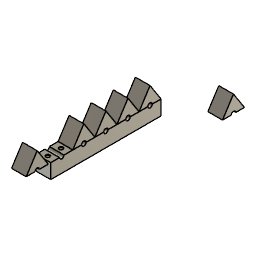
cabel organizer prototype (Autodesk Fusion 360 archive; units mm, degrees)
design "eg project work"
part number: 2025-11-05-01-47-41-680
Autodesk Fusion 360 part; units mm, degrees
sketch "Sketch1" plane through (0, 0, 0) normal (1, 0, 0) x (0, 1, 0)
  line L0 (-100, 50) -> (125, 50)
  line L1 (125, 50) -> (125, 20)
  line L2 (-100, 50) -> (-100, 20)
  line L3 (-100, 20) -> (125, 20)
  dimension "d1" = 225
  dimension "d2" = 30
  dimension "d3" = 30
  constraint horizontal L0
  constraint perpendicular L0 L1
  constraint perpendicular L0 L2
  measures "d1" distance of L0.start L0.end
  measures "d2" distance of L0.end L1.end
  measures "d3" distance of L0.start L2.end
extrude "Extrude1" add sketch "Sketch1" along normal blind 30 makes body 1
sketch "Sketch2" plane through (30, 0, 0) normal (1, 0, 0) x (0, 1, 0)
  line L0 (-100, 50) -> (-100, 20)
  line L1 (-100, 20) -> (125, 20)
  line L2 (125, 20) -> (125, 50)
  line L3 (125, 50) -> (-100, 50)
  circle A0 centre (-91, 50) radius 4
  line L4 (-87, 50) -> (-82, 50)
  circle A1 centre (-77.5, 50) radius 4.5
  line L5 (-73, 50) -> (-68, 50)
  circle A2 centre (-64, 50) radius 4
  line L6 (-60, 50) -> (-50, 50)
  circle A3 centre (-46, 50) radius 4
  line L7 (-42, 50) -> (-37, 50)
  circle A4 centre (-32.5, 50) radius 4.5
  line L8 (-28, 50) -> (-23, 50)
  circle A5 centre (-19.0025, 49.8588) radius 4
  line L9 (-15.005, 50) -> (-5.005, 50)
  circle A6 centre (-1.005, 50) radius 4
  line L10 (2.995, 50) -> (7.995, 50)
  circle A7 centre (12.495, 50) radius 4.5
  line L11 (16.995, 50) -> (21.995, 50)
  circle A8 centre (25.995, 50) radius 4
  line L12 (29.995, 50) -> (34.995, 50)
  line L13 (34.995, 50) -> (39.995, 50)
  circle A9 centre (43.995, 50) radius 4
  line L14 (47.995, 50) -> (52.995, 50)
  circle A10 centre (57.495, 50) radius 4.5
  line L15 (61.995, 50) -> (66.995, 50)
  circle A11 centre (70.995, 50) radius 4
  line L16 (74.995, 50) -> (79.995, 50)
  line L17 (79.995, 50) -> (84.995, 50)
  circle A12 centre (88.995, 50) radius 4
  line L18 (92.995, 50) -> (97.995, 50)
  circle A13 centre (102.495, 50) radius 4.5
  line L19 (106.995, 50) -> (111.995, 50)
  circle A14 centre (115.995, 50) radius 4
  dimension "d6" = 8
  dimension "d7" = 5
  dimension "d8" = 9
  dimension "d9" = 5
  dimension "d10" = 8
  dimension "d11" = 10
  dimension "d12" = 8
  dimension "d13" = 5
  dimension "d14" = 9
  dimension "d15" = 5
  dimension "d16" = 8
  dimension "d17" = 10
  dimension "d18" = 8
  dimension "d19" = 5
  dimension "d20" = 9
  dimension "d21" = 5
  dimension "d22" = 8
  dimension "d23" = 5
  dimension "d24" = 5
  dimension "d25" = 8
  dimension "d26" = 5
  dimension "d27" = 9
  dimension "d28" = 5
  dimension "d29" = 8
  dimension "d30" = 5
  dimension "d31" = 5
  dimension "d32" = 8
  dimension "d33" = 5
  dimension "d34" = 9
  dimension "d35" = 5
  dimension "d36" = 8
  constraint coincident A0 L4.start
  constraint coincident L3 L4.start
  constraint perpendicular L0 L4
  constraint coincident L4.end A1
  constraint coincident A1 L5.start
  constraint coincident L3 L5.start
  constraint parallel L3 L5
  constraint coincident L5.end A2
  constraint coincident A2 L6.start
  constraint coincident L3 L6.start
  constraint parallel L3 L6
  constraint coincident L6.end A3
  constraint coincident L3 L7.start
  constraint coincident A3 L7.start
  constraint parallel L3 L7
  constraint coincident L7.end A4
  constraint coincident A4 L8.start
  constraint coincident L3 L8.start
  constraint parallel L3 L8
  constraint coincident L8.end A5
  constraint coincident A5 L9.start
  constraint coincident L3 L9.start
  constraint parallel L3 L9
  constraint coincident L9.end A6
  constraint coincident A6 L10.start
  constraint coincident L3 L10.start
  constraint parallel L3 L10
  constraint coincident L10.end A7
  constraint coincident A7 L11.start
  constraint coincident L3 L11.start
  constraint parallel L3 L11
  constraint coincident L11.end A8
  constraint coincident A8 L12.start
  constraint coincident L3 L12.start
  constraint parallel L3 L12
  constraint parallel L3 L13
  constraint coincident L13.end A9
  constraint coincident A9 L14.start
  constraint coincident L3 L14.start
  constraint parallel L3 L14
  constraint coincident L14.end A10
  constraint coincident A10 L15.start
  constraint coincident L3 L15.start
  constraint parallel L3 L15
  constraint coincident L15.end A11
  constraint coincident A11 L16.start
  constraint coincident L3 L16.start
  constraint coincident L3 L16.end
  constraint parallel L3 L17
  constraint coincident L17.end A12
  constraint coincident A12 L18.start
  constraint coincident L3 L18.start
  constraint parallel L3 L18
  constraint coincident L18.end A13
  constraint coincident A13 L19.start
  constraint coincident L3 L19.start
  constraint coincident L3 L19.end
  constraint coincident L19.end A14
  measures "d6" diameter of A0
  measures "d7" distance of L4.start L4.end
  measures "d8" diameter of A1
  measures "d9" distance of L5.start L5.end
  measures "d10" diameter of A2
  measures "d11" distance of L6.start L6.end
  measures "d12" diameter of A3
  measures "d13" distance of L7.start L7.end
  measures "d14" diameter of A4
  measures "d15" distance of L8.start L8.end
  measures "d16" diameter of A5
  measures "d17" distance of L9.start L9.end
  measures "d18" diameter of A6
  measures "d19" distance of L10.start L10.end
  measures "d20" diameter of A7
  measures "d21" distance of L11.start L11.end
  measures "d22" diameter of A8
  measures "d23" distance of L12.start L12.end
  measures "d24" distance of L12.end L13.end
  measures "d25" diameter of A9
  measures "d26" distance of L14.start L14.end
  measures "d27" diameter of A10
  measures "d28" distance of L15.start L15.end
  measures "d29" diameter of A11
  measures "d30" distance of L16.start L16.end
  measures "d31" distance of L16.end L17.end
  measures "d32" diameter of A12
  measures "d33" distance of L18.start L18.end
  measures "d34" diameter of A13
  measures "d35" distance of L19.start L19.end
  measures "d36" diameter of A14
extrude "Extrude2" cut sketch "Sketch2" against normal blind 30 contours L3 A1 | L3 A13 | L3 A4 | L3 A10 | L3 A7 picked at (-78.5177, 47.8868) picked at (102.2431, 47.4446) picked at (-32.3879, 47.6199) picked at (56.1436, 48.902) picked at (11.6784, 48.2588) bodies 1
sketch "Sketch3" plane through (0, 0, 50) normal (0, 0, 1) x (-1, 0, 0)
  line L0 (-30, 82) -> (0, 82)
  line L1 (0, 82) -> (0, 100)
  line L2 (0, 100) -> (-30, 100)
  line L3 (-30, 100) -> (-30, 82)
  circle A0 centre (-15, 91) radius 4
  circle A1 centre (-15, 64) radius 4
  circle A2 centre (-15, 46) radius 4
  circle A3 centre (-15, 19) radius 4
  circle A4 centre (-14.9699, 1.0001) radius 4
  circle A5 centre (-15, -26) radius 4
  circle A6 centre (-15, -44) radius 4
  circle A7 centre (-14.9455, -70.9996) radius 4
  circle A8 centre (-15, -89) radius 4
  circle A9 centre (-15, -116) radius 4
  dimension "d39" = 8
  dimension "d40" = 8
  dimension "d41" = 8
  dimension "d42" = 8
  dimension "d43" = 8
  dimension "d44" = 8
  dimension "d45" = 8
  dimension "d46" = 8
  dimension "d47" = 8
  dimension "d48" = 8
  measures "d39" diameter of A0
  measures "d40" diameter of A1
  measures "d41" diameter of A2
  measures "d42" diameter of A3
  measures "d43" diameter of A4
  measures "d44" diameter of A5
  measures "d45" diameter of A6
  measures "d46" diameter of A7
  measures "d47" diameter of A8
  measures "d48" diameter of A9
extrude "Extrude3" cut sketch "Sketch3" against normal blind 1.5 contours A0 | A1 | A2 | A3 | A4 | A5 | A6 | A7 | A8 | A9 bodies 1
sketch "Sketch4" plane through (0, 0, 0) normal (1, 0, 0) x (0, 1, 0)
  line L0 (50, -50) -> (95, -50)
  line L1 (72.5, -50) -> (72.5, -15)
  line L2 (72.5, -15) -> (50, -50)
  line L3 (72.5, -15) -> (95, -50)
  constraint horizontal L0
  constraint midpoint L0 L1.start
  constraint perpendicular L0 L1
extrude "Extrude4" add sketch "Sketch4" along normal blind 30 separate body makes body 2
sketch "Sketch5" plane through (30, 0, 0) normal (1, 0, 0) x (0, 1, 0)
  line L0 (50, -50) -> (95, -50)
  line L1 (95, -50) -> (72.5, -15)
  line L2 (72.5, -15) -> (50, -50)
  circle A0 centre (72.5, -50) radius 4.5
  line L3 (77, -50) -> (82, -50)
  dimension "d53" = 9
  dimension "d54" = 5
  constraint midpoint L0 A0.centre
  constraint coincident A0 L3.start
  constraint coincident L0 L3.start
  constraint parallel L0 L3
  measures "d53" diameter of A0
  measures "d54" distance of L3.start L3.end
extrude "Extrude5" add sketch "Sketch5" along normal blind 30 contours L0 A0 picked at (72.1662, -48.5376) bodies 2
extrude "Extrude6" cut 1 faces at (60, 72.1662, -48.5376) along direction (-1, 0, 0) blind 60 on bodies 2 bodies 2
sketch "Sketch6" plane through (0, 0, -50) normal (0, 0, -1) x (1, 0, 0)
  line L0 (0, -68) -> (30, -68)
  line L1 (30, -68) -> (30, -50)
  line L2 (30, -50) -> (0, -50)
  line L3 (0, -50) -> (0, -68)
  circle A0 centre (14.9693, -58.9999) radius 4
  circle A1 centre (15, -86) radius 4
  dimension "d59" = 8
  dimension "d60" = 8
  measures "d59" diameter of A0
  measures "d60" diameter of A1
extrude "Extrude7" cut sketch "Sketch6" against normal blind 1.5 contours A0 | A1 bodies 2
copy_body "CopyPasteBodies1" bodies 2 makes body 3
move_body "Move1" bodies 3 to x (1, 0, 0) y (0, 1, 0) z (0, 0, 1) at (0, 0, 150)
copy_body "CopyPasteBodies2" bodies 2 makes body 4
move_body "Move2" bodies 4 to x (1, 0, 0) y (0, 1, 0) z (0, 0, 1) at (0, 125, 0)
copy_body "CopyPasteBodies3" bodies 2 makes body 5
move_body "Move3" bodies 5 to x (1, 0, 0) y (0, 1, 0) z (0, 0, 1) at (0, 0, 225)
copy_body "CopyPasteBodies4" bodies 2 makes body 6
copy_body "CopyPasteBodies5" bodies 2 makes body 7
move_body "Move4" bodies 7 to x (1, 0, 0) y (0, 1, 0) z (0, 0, 1) at (0, 200, 0)
move_body "Move5" bodies 6 2 to x (1, 0, 0) y (0, 1, 0) z (0, 0, 1) at (0, 30, 100)
move_body "Move6" bodies 3 to x (1, 0, 0) y (0, 1, 0) z (0, 0, 1) at (0, -15, -50)
move_body "Move7" bodies 4 to x (1, 0, 0) y (0, 1, 0) z (0, 0, 1) at (0, -185, 100)
move_body "Move8" bodies 5 to x (1, 0, 0) y (0, 1, 0) z (0, 0, 1) at (0, -105, -125)
copy_body "CopyPasteBodies6" bodies 2 makes body 8
move_body "Move10" bodies 8 to x (1, 0, 0) y (0, 1, 0) z (0, 0, 1) at (0, -230, 0)
